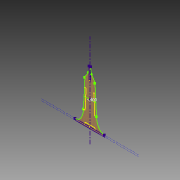
# Autodesk Inventor part: Bottom Plate v2
Saved by Autodesk Inventor 2013 SP1 (Build 170176100, 176)
## iProperties
Created: 2013-02-28
Part Number: Bottom Plate v2
Material: Wood (Cherry)
Document SubType Name: Modeling
Designer: fixer
Mass: 59.0239 g
Surface Area: 779.579 cm^2
Volume: 118.048 cm^3
Density: 0.5 g/cm^3
Author: fixer
Autodesk Inventor part; units mm, degrees
ref_plane "YZ Plane" through (0, 0, 0) normal (1, 0, 0) x (0, 1, 0)
ref_plane "XZ Plane" through (0, 0, 0) normal (0, 1, 0) x (-1, 0, 0)
ref_plane "XY Plane" through (0, 0, 0) normal (0, 0, 1) x (1, 0, 0)
sketch "Sketch1" plane through (0, 0, 0) normal (0, 0, 1) x (1, 0, 0)
  line L0 (76.2, -12.7) -> (381, -12.7) construction
  line L1 (-76.2, -12.7) -> (-381, -12.7) construction
  line L2 (-76.2, 0) -> (-381, 0) construction
  line L3 (76.2, 0) -> (381, 0) construction
  line L4 (0, -116.2267) -> (0, 608.4603)
  line L5 (0, -12.7) -> (-114.3, -12.7)
  line L6 (-114.3, -12.7) -> (-114.3, 0)
  line L7 (0, 406.4) -> (-6.35, 406.4)
  line L8 (-39.0138, 312.42) -> (-50.5988, 93.6374)
  line L9 (39.0138, 312.42) -> (50.5988, 93.6374)
  line L10 (0, 406.4) -> (6.35, 406.4)
  line L11 (0, -12.7) -> (114.3, -12.7)
  line L12 (114.3, -12.7) -> (114.3, 0)
  spline S0 degree 4 poles (-6.35, 406.4) (-6.35, 381.154) (-10.7035, 365.7003) (-9.9482, 354.3709) (-38.2791, 326.2946) (-39.0138, 312.42) knots 0 0 0 0 0 0.492384 1 1 1 1 1
  line L13 (-6.35, 441.1174) -> (-6.35, 371.6826) construction
  arc A0 (-7.3193, 378.694) -> (-7.3193, 434.106) centre (-402.7904, 406.4) ccw construction
  spline S1 degree 4 poles (6.35, 406.4) (6.35, 381.154) (10.7035, 365.7003) (9.9482, 354.3709) (38.2791, 326.2946) (39.0138, 312.42) knots 0 0 0 0 0 0.492384 1 1 1 1 1
  line L14 (6.35, 441.1174) -> (6.35, 371.6826) construction
  arc A1 (7.3193, 434.106) -> (7.3193, 378.694) centre (402.7904, 406.4) ccw construction
  line L15 (-8.1247, 369.9755) -> (-17.7136, 348.6922) construction
  arc A2 (-17.4133, 351.2643) -> (-9.8522, 368.0464) centre (-62.6107, 381.7218) ccw construction
  line L16 (8.1247, 369.9755) -> (17.7136, 348.6922) construction
  arc A3 (9.8522, 368.0464) -> (17.4133, 351.2643) centre (62.6107, 381.7218) ccw construction
  spline S2 degree 3 poles (-50.5988, 93.6374) (-52.7393, 53.2143) (-67.314, 0) (-114.3, 0) knots 0 0 0 0 1 1 1 1
  line L17 (-100.9407, 0) -> (-127.6593, 0) construction
  arc A4 (-124.8332, 0.8979) -> (-103.7668, 0.8979) centre (-114.3, 62.2299) ccw construction
  spline S3 degree 3 poles (50.5988, 93.6374) (52.7393, 53.2143) (67.314, 0) (114.3, 0) knots 0 0 0 0 1 1 1 1
  line L18 (100.9407, 0) -> (127.6593, 0) construction
  arc A5 (103.7668, 0.8979) -> (124.8332, 0.8979) centre (114.3, 62.2299) ccw construction
  point P0 (0, 0)
  point P1 (-12.9192, 359.3339)
  point P2 (12.9192, 359.3339)
  dimension "d3" = 114.3
  dimension "d5" = 0.7
  dimension "d6" = 0.7
  dimension "d7" = 93.98
  dimension "d8" = 12.7
  dimension "d9" = 419.1
  constraints: 38 end point, 15 symmetric about line, 10 midpoint, 9 horizontal, 6 centre point, 6 point on circle, 5 point on line, 4 vertical, 2 perpendicular, 25 other
  measures "d3" distance of L5.start L11.end
  measures "d7" distance from line of L9.start L10
  measures "d8" diameter of L10.end L4
  measures "d9" distance between parallel lines of L10 L11
extrude "Extrusion1" add sketch "Sketch1" against normal blind 3.175
sketch "Etching" plane through (0, 0, 0) normal (0, 0, 1) x (1, 0, 0)
  line L0 (-114.3, -12.7) -> (114.3, -12.7) projected
  line L1 (114.3, -12.7) -> (114.3, 0) projected
  line L2 (50.5988, 93.6374) -> (39.0138, 312.42) projected
  line L3 (6.35, 406.4) -> (-6.35, 406.4) projected
  line L4 (-39.0138, 312.42) -> (-50.5988, 93.6374) projected
  line L5 (-114.3, 0) -> (-114.3, -12.7) projected
  line L6 (-45.7985, 184.2911) -> (45.7985, 184.2911)
  line L7 (0, -12.7) -> (0, 406.4)
  circle A0 centre (0, 184.2911) radius 5.08
  line L8 (-38.1, 12.7) -> (38.1, 12.7) projected
  line L9 (-38.1, 0) -> (-38.1, 12.7) projected
  line L10 (38.1, 12.7) -> (38.1, 0) projected
  line L11 (-114.3, 0) -> (114.3, 0)
  line L12 (37.9166, 92.9659) -> (29.8579, 245.1527) projected
  line L13 (42.5402, 245.8242) -> (29.8579, 245.1527) projected
  line L14 (37.9166, 92.9659) -> (50.5988, 93.6374) projected
  line L15 (-50.5988, 93.6374) -> (-37.9166, 92.9659) projected
  line L16 (-37.9166, 92.9659) -> (-29.8579, 245.1527) projected
  line L17 (-29.8579, 245.1527) -> (-42.5402, 245.8242) projected
  line L18 (-6.35, 298.8732) -> (6.35, 298.8732) projected
  line L19 (-6.35, 298.8732) -> (-6.35, 406.4)
  line L20 (6.35, 298.8732) -> (6.35, 406.4)
  dimension "d10" = 10.16
  constraints: 10 end point, 3 perpendicular, 2 midpoint, 2 point on line, 1 centre point, 1 coincident, 1 parallel, 4 other
  measures "d10" diameter of A0
equation "\"d5\" = d6"
body "Solid1"
